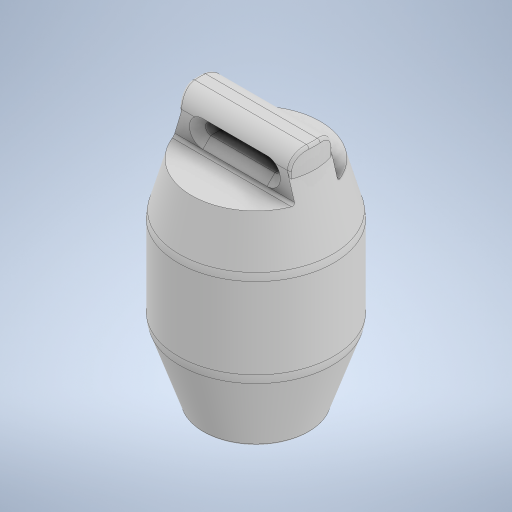
# Autodesk Inventor part: paddle_end
Saved by Autodesk Inventor 2023.4 (Build 274418000, 418)
## iProperties
Created: 2024-02-17
Part Number: paddle_end
Material: Generic
Document SubType Name: Modeling
Designer: aaron
Density: 1 g/cm^3
Appearance: Default
Author: aaron
Autodesk Inventor part; units mm, degrees
ref_plane "YZ Plane" through (0, 0, 0) normal (1, 0, 0) x (0, 1, 0)
ref_plane "XZ Plane" through (0, 0, 0) normal (0, 1, 0) x (-1, 0, 0)
ref_plane "XY Plane" through (0, 0, 0) normal (0, 0, 1) x (1, 0, 0)
sketch "Sketch1" plane through (0, 0, 0) normal (0, 0, 1) x (1, 0, 0)
  line L0 (14, 0) -> (14, 49.25)
  line L1 (14, 49.25) -> (21.05, 49.25)
  line L2 (21.05, 49.25) -> (21.05, 41.2)
  line L3 (21.05, 41.2) -> (14, 41.2)
  line L4 (14, 41.2) -> (14, 77.25)
  line L5 (14, 77.25) -> (0, 79.25)
  line L6 (0, 79.25) -> (0, 95.25)
  line L7 (0, 95.25) -> (21.05, 82.4891)
  line L8 (21.05, 82.4891) -> (29.05, 61.25)
  line L9 (29.05, 61.25) -> (29.05, 28)
  line L10 (29.05, 28) -> (19.5584, 0)
  line L11 (19.5584, 0) -> (14, 0)
  line L12 (0, 95.25) -> (22, 95.25)
  line L13 (22, 95.25) -> (22, 86.6164)
  line L14 (22, 86.6164) -> (29.05, 61.25)
  point P0 (0, 0)
  point P1 (5.988, 122.4768)
  point P2 (14, 49.25)
  dimension "d0" = 7.05
  dimension "d2" = 0
  dimension "d3" = 14
  dimension "d4" = 0
  dimension "d6" = 8.05
  dimension "d7" = 2
  dimension "d8" = 16
  dimension "d9" = 28
  dimension "d10" = 16
  dimension "d11" = 8
  dimension "d12" = 22
  dimension "d43" = 28
  dimension "d44" = 41.2
  constraints: 30 end point, 4 point on line, 3 parallel, 3 perpendicular, 2 vertical, 1 horizontal
  measures "d0" distance of L0.end L1.end
  measures "d2" distance from line of point (0, 0) L11
  measures "d3" distance from line of point (0, 0) L0
  measures "d4" distance from line of point (0, 0) L6
  measures "d6" distance of L1.end L2.end
  measures "d7" vertical distance of L5.end L4.end
  measures "d8" distance of L5.end L6.end
  measures "d9" distance from line of L11 L9.end
  measures "d10" vertical distance of L8.end L4.end
  measures "d11" distance between parallel lines of L2 L9
  measures "d12" distance of L6.end L12.end
  measures "d43" distance from line of L4.end L1
  measures "d44" distance from line of L0.start L3
revolve "Revolution1" add sketch "Sketch1" angle 360 about axis through (0, 79.25, 0) along (0, 1, 0) contours L0 L3 L2 L1 L4 L5 L6 L7 L8 L9 L10 L11 | L8 L7 L12 L13 L14
sketch "Sketch2" plane through (0, 95.25, 0) normal (0, 1, 0) x (1, 0, 0)
  line L0 (-33.2869, 8) -> (36.0834, 8)
  line L1 (36.0834, 8) -> (36.0834, 35.7842)
  line L2 (36.0834, 35.7842) -> (-33.2869, 35.7842)
  line L3 (-33.2869, 35.7842) -> (-33.2869, 8)
  line L4 (38.7896, -8) -> (-41.3154, -8)
  line L5 (-41.3154, -8) -> (-41.3154, -27.9361)
  line L6 (-41.3154, -27.9361) -> (38.7896, -27.9361)
  line L7 (38.7896, -27.9361) -> (38.7896, -8)
  point P0 (0, 0)
  dimension "d14" = 8
  dimension "d15" = 8
  constraints: 16 end point, 4 parallel, 2 horizontal, 2 perpendicular
  measures "d14" distance from line of L0 point (0, 0)
  measures "d15" distance from line of point (0, 0) L4
extrude "Extrusion1" cut sketch "Sketch2" against normal blind 16
sketch "Sketch3" plane through (-20.4939, 95.25, 8) normal (0, 0, 1) x (1, 0, 0)
  line L0 (6.6018, -8) -> (34.6018, -8)
  line L1 (34.6018, -8) -> (34.6018, -12)
  line L2 (34.6018, -12) -> (6.6018, -12)
  line L3 (6.6018, -12) -> (6.6018, -8)
  line L4 (6.6018, -10) -> (0.2158, -10)
  line L5 (34.6018, -10) -> (40.9878, -10)
  line L6 (40.9878, 0) -> (40.9878, -8.6336) projected
  line L7 (0, 0) -> (40.9878, 0) projected
  point P0 (20.4939, -95.25)
  point P1 (40.9878, -15.8903)
  dimension "d18" = 28
  dimension "d19" = 4
  dimension "d20" = 8
  constraints: 12 end point, 3 horizontal, 2 midpoint, 2 parallel, 1 collinear, 1 perpendicular, 1 point on line
  measures "d18" distance of L0.start L0.end
  measures "d19" distance between parallel lines of L2 L0
  measures "d20" distance between parallel lines of L7 L0
extrude "Extrusion2" cut sketch "Sketch3" against normal through all
fillet "Fillet1" radius 2 4 edges at (-13.8921, 87.25, 0) (-13.8921, 83.25, 0) (14.1079, 87.25, 0) (14.1079, 83.25, 0)
chamfer "Chamfer1" distance 3 angle 45 16 edges at (0.1079, 87.25, 8) (13.5221, 86.6642, 8) (14.1079, 85.25, 8) (13.5221, 83.8358, 8) (0.1079, 83.25, 8) (-13.3063, 86.6642, 8) (-13.8921, 85.25, 8) (-13.3063, 83.8358, 8) (0.1079, 87.25, -8) (-13.3063, 86.6642, -8) (-13.8921, 85.25, -8) (-13.3063, 83.8358, -8) (0.1079, 83.25, -8) (13.5221, 86.6642, -8) (14.1079, 85.25, -8) (13.5221, 83.8358, -8)
fillet "Fillet2" radius 6 2 edges at (0, 95.25, 8) (0, 95.25, -8)
fillet "Fillet3" radius 1 12 edges at (0, 79.25, 8) (0, 79.25, -8) (-22, 95.25, 0) (-21.0019, 93.1598, 6.5512) (-20.4939, 87.9332, 8) (-20.4939, 87.9332, -8) (-21.0012, 93.157, -6.5536) (22, 95.25, 0) (21.0012, 93.157, -6.5536) (20.4939, 87.9332, -8) (20.4939, 87.9332, 8) (20.9975, 93.1431, 6.5655)
fillet "Fillet4" radius 10 2 edges at (-29.05, 61.25, 0) (-29.05, 28, 0)
chamfer "Chamfer2" distance 1 angle 45 1 edges at (-14, 0, 0)
sketch "Sketch4" plane through (19.3806, 64.15, -8) normal (0, 0, -1) x (-1, 0, 0)
  line L0 (40.4306, -22.95) -> (-1.6694, -22.95) projected
  line L1 (-1.6694, -14.9) -> (-1.6694, -22.95) projected
  line L2 (40.4306, -14.9) -> (-1.6694, -14.9) projected
  line L3 (40.4306, -14.9) -> (40.4306, -22.95) projected
  circle A0 centre (18.6514, -18.925) radius 4.025
  circle A1 centre (18.6514, -18.925) radius 4.525
  point P0 (19.3806, -64.15)
  dimension "d35" = 0.5
  constraints: 2 centre point, 2 tangent
  measures "d35" radial gap between concentric circles of A0 A1
extrude "Extrusion3" cut sketch "Sketch4" along normal blind 30.6 contours A1 L0 | L0 A0 L2 A1 | L0 A1 L2 A0 | A0 | L2 A1
chamfer "Chamfer3" distance 4 angle 45 1 edges at (5.2524, 45.3502, -28.5712)
fillet "Fillet5" radius 1 1 edges at (-19.5584, 0, 0)
chamfer "Chamfer4" distance 0.5 angle 45 6 edges at (-9.4144, 49.25, 10.3619) (10.8433, 49.25, -8.8556) (-9.4144, 41.2, 10.3619) (10.8433, 41.2, -8.8556) (-0.7327, 49.25, 21.0372) (-0.7327, 41.2, 21.0372)
equation "\"d15\" = d14"
body "Solid1"
